Autodesk Inventor part; units mm, degrees
(part 13 of 13)
  line L4684 (16.4485, 3.9123) -> (16.4485, 3.1666)
  arc A4680 (16.4485, 3.1666) -> (16.6009, 3.1666) centre (16.5247, 3.1666) ccw
  line L4685 (16.6009, 3.1666) -> (16.6009, 3.9123)
  arc A4681 (16.6009, 3.9123) -> (16.4485, 3.9123) centre (16.5247, 3.9123) ccw
  line L4686 (16.5247, 3.2428) -> (15.9654, 3.2428)
  arc A4682 (15.9654, 3.2428) -> (15.9654, 3.0904) centre (15.9654, 3.1666) ccw
  line L4687 (15.9654, 3.0904) -> (16.5247, 3.0904)
  arc A4683 (16.5247, 3.0904) -> (16.5247, 3.2428) centre (16.5247, 3.1666) ccw
  line L4688 (16.0335, 3.1325) -> (16.22, 3.5053)
  arc A4684 (16.22, 3.5053) -> (16.0838, 3.5735) centre (16.1519, 3.5394) ccw
  line L4689 (16.0838, 3.5735) -> (15.8973, 3.2007)
  arc A4685 (15.8973, 3.2007) -> (16.0335, 3.1325) centre (15.9654, 3.1666) ccw
  line L4690 (16.2281, 3.5394) -> (16.2281, 3.7258)
  arc A4686 (16.2281, 3.7258) -> (16.0757, 3.7258) centre (16.1519, 3.7258) ccw
  line L4691 (16.0757, 3.7258) -> (16.0757, 3.5394)
  arc A4687 (16.0757, 3.5394) -> (16.2281, 3.5394) centre (16.1519, 3.5394) ccw
  line L4692 (16.2058, 3.7797) -> (16.0193, 3.9662)
  arc A4688 (16.0193, 3.9662) -> (15.9115, 3.8584) centre (15.9654, 3.9123) ccw
  line L4693 (15.9115, 3.8584) -> (16.098, 3.6719)
  arc A4689 (16.098, 3.6719) -> (16.2058, 3.7797) centre (16.1519, 3.7258) ccw
  line L4694 (15.9654, 3.9885) -> (15.5926, 3.9885)
  arc A4690 (15.5926, 3.9885) -> (15.5926, 3.8361) centre (15.5926, 3.9123) ccw
  line L4695 (15.5926, 3.8361) -> (15.9654, 3.8361)
  arc A4691 (15.9654, 3.8361) -> (15.9654, 3.9885) centre (15.9654, 3.9123) ccw
  line L4696 (15.5387, 3.9662) -> (15.3523, 3.7797)
  arc A4692 (15.3523, 3.7797) -> (15.4601, 3.6719) centre (15.4062, 3.7258) ccw
  line L4697 (15.4601, 3.6719) -> (15.6465, 3.8584)
  arc A4693 (15.6465, 3.8584) -> (15.5387, 3.9662) centre (15.5926, 3.9123) ccw
  line L4698 (15.33, 3.7258) -> (15.33, 3.353)
  arc A4694 (15.33, 3.353) -> (15.4824, 3.353) centre (15.4062, 3.353) ccw
  line L4699 (15.4824, 3.353) -> (15.4824, 3.7258)
  arc A4695 (15.4824, 3.7258) -> (15.33, 3.7258) centre (15.4062, 3.7258) ccw
  line L4700 (15.3523, 3.2991) -> (15.5387, 3.1127)
  arc A4696 (15.5387, 3.1127) -> (15.6465, 3.2205) centre (15.5926, 3.1666) ccw
  line L4701 (15.6465, 3.2205) -> (15.4601, 3.4069)
  arc A4697 (15.4601, 3.4069) -> (15.3523, 3.2991) centre (15.4062, 3.353) ccw
  line L4702 (15.4062, 4.2597) -> (16.5247, 4.2597)
  arc A4698 (16.5247, 4.2597) -> (16.5247, 4.4121) centre (16.5247, 4.3359) ccw
  line L4703 (16.5247, 4.4121) -> (15.4062, 4.4121)
  arc A4699 (15.4062, 4.4121) -> (15.4062, 4.2597) centre (15.4062, 4.3359) ccw
  line L4704 (16.5786, 4.3898) -> (16.2058, 4.7626)
  arc A4700 (16.2058, 4.7626) -> (16.098, 4.6548) centre (16.1519, 4.7087) ccw
  line L4705 (16.098, 4.6548) -> (16.4708, 4.282)
  arc A4701 (16.4708, 4.282) -> (16.5786, 4.3898) centre (16.5247, 4.3359) ccw
  line L4706 (16.2058, 4.6548) -> (16.5786, 5.0277)
  arc A4702 (16.5786, 5.0277) -> (16.4708, 5.1355) centre (16.5247, 5.0816) ccw
  line L4707 (16.4708, 5.1355) -> (16.098, 4.7626)
  arc A4703 (16.098, 4.7626) -> (16.2058, 4.6548) centre (16.1519, 4.7087) ccw
  arc A4704 (3.9356, 63.3973) -> (3.8278, 63.5051) centre (3.8817, 63.4512) ccw
  line L4708 (3.8278, 63.5051) -> (3.6414, 63.3186)
  arc A4705 (3.6414, 63.3186) -> (3.7492, 63.2108) centre (3.6953, 63.2647) ccw
  line L4709 (3.8817, 63.375) -> (4.0681, 63.375)
  arc A4706 (4.0681, 63.375) -> (4.0681, 63.5274) centre (4.0681, 63.4512) ccw
  line L4710 (4.0681, 63.5274) -> (3.8817, 63.5274)
  arc A4707 (3.8817, 63.5274) -> (3.8817, 63.375) centre (3.8817, 63.4512) ccw
  line L4711 (4.0142, 63.3973) -> (4.2007, 63.2108)
  arc A4708 (4.2007, 63.2108) -> (4.3085, 63.3186) centre (4.2546, 63.2647) ccw
  line L4712 (4.3085, 63.3186) -> (4.122, 63.5051)
  arc A4709 (4.122, 63.5051) -> (4.0142, 63.3973) centre (4.0681, 63.4512) ccw
  arc A4710 (2.9, 16.9912) -> (2.7476, 16.9912) centre (2.8238, 16.9912) ccw
  arc A4711 (4.1784, 63.0783) -> (4.3308, 63.0783) centre (4.2546, 63.0783) ccw
  line L4713 (4.3308, 63.0783) -> (4.3308, 63.2647)
  arc A4712 (4.3308, 63.2647) -> (4.1784, 63.2647) centre (4.2546, 63.2647) ccw
  line L4714 (4.3085, 63.2108) -> (4.4949, 63.3973)
  arc A4713 (4.4949, 63.3973) -> (4.3871, 63.5051) centre (4.441, 63.4512) ccw
  line L4715 (4.3871, 63.5051) -> (4.2007, 63.3186)
  arc A4714 (4.2007, 63.3186) -> (4.3085, 63.2108) centre (4.2546, 63.2647) ccw
  line L4716 (4.441, 63.375) -> (4.6274, 63.375)
  arc A4715 (4.6274, 63.375) -> (4.6274, 63.5274) centre (4.6274, 63.4512) ccw
  line L4717 (4.6274, 63.5274) -> (4.441, 63.5274)
  arc A4716 (4.441, 63.5274) -> (4.441, 63.375) centre (4.441, 63.4512) ccw
  line L4718 (4.5735, 63.3973) -> (4.7599, 63.2108)
  arc A4717 (4.7599, 63.2108) -> (4.8677, 63.3186) centre (4.8138, 63.2647) ccw
  line L4719 (4.8677, 63.3186) -> (4.6813, 63.5051)
  arc A4718 (4.6813, 63.5051) -> (4.5735, 63.3973) centre (4.6274, 63.4512) ccw
  line L4720 (4.1784, 63.2647) -> (4.1784, 63.0783)
  line L4721 (4.7376, 63.2647) -> (4.7376, 62.8919)
  arc A4719 (4.7376, 62.8919) -> (4.89, 62.8919) centre (4.8138, 62.8919) ccw
  line L4722 (4.89, 62.8919) -> (4.89, 63.2647)
  arc A4720 (4.89, 63.2647) -> (4.7376, 63.2647) centre (4.8138, 63.2647) ccw
  line L4723 (4.7599, 62.9458) -> (4.5735, 62.7594)
  arc A4721 (4.5735, 62.7594) -> (4.6813, 62.6516) centre (4.6274, 62.7055) ccw
  line L4724 (4.6813, 62.6516) -> (4.8677, 62.838)
  arc A4722 (4.8677, 62.838) -> (4.7599, 62.9458) centre (4.8138, 62.8919) ccw
  line L4725 (2.6913, 15.0223) -> (2.8777, 15.2087)
  arc A4723 (2.8777, 15.2087) -> (2.7699, 15.3165) centre (2.8238, 15.2626) ccw
  line L4726 (2.7699, 15.3165) -> (2.5835, 15.1301)
  arc A4724 (2.5835, 15.1301) -> (2.6913, 15.0223) centre (2.6374, 15.0762) ccw
  line L4727 (2.9, 15.2626) -> (2.9, 15.449)
  arc A4725 (2.9, 15.449) -> (2.7476, 15.449) centre (2.8238, 15.449) ccw
  line L4728 (2.7476, 15.449) -> (2.7476, 15.2626)
  arc A4726 (2.7476, 15.2626) -> (2.9, 15.2626) centre (2.8238, 15.2626) ccw
  line L4729 (2.8777, 15.5029) -> (2.6913, 15.6893)
  arc A4727 (2.6913, 15.6893) -> (2.5835, 15.5815) centre (2.6374, 15.6354) ccw
  line L4730 (2.5835, 15.5815) -> (2.7699, 15.3951)
  arc A4728 (2.7699, 15.3951) -> (2.8777, 15.5029) centre (2.8238, 15.449) ccw
  line L4731 (2.6374, 15.7116) -> (1.7053, 15.7116)
  arc A4729 (1.7053, 15.7116) -> (1.7053, 15.5592) centre (1.7053, 15.6354) ccw
  line L4732 (1.7053, 15.5592) -> (2.6374, 15.5592)
  arc A4730 (2.6374, 15.5592) -> (2.6374, 15.7116) centre (2.6374, 15.6354) ccw
  line L4733 (1.7815, 15.449) -> (1.7815, 15.8219)
  arc A4731 (1.7815, 15.8219) -> (1.6291, 15.8219) centre (1.7053, 15.8219) ccw
  line L4734 (1.6291, 15.8219) -> (1.6291, 15.449)
  arc A4732 (1.6291, 15.449) -> (1.7815, 15.449) centre (1.7053, 15.449) ccw
  line L4735 (2.132, 16.2994) -> (1.7592, 16.6722)
  arc A4733 (1.7592, 16.6722) -> (1.6514, 16.5644) centre (1.7053, 16.6183) ccw
  line L4736 (1.6514, 16.5644) -> (2.0242, 16.1916)
  arc A4734 (2.0242, 16.1916) -> (2.132, 16.2994) centre (2.0781, 16.2455) ccw
  line L4737 (1.7053, 16.5421) -> (2.8238, 16.5421)
  arc A4735 (2.8238, 16.5421) -> (2.8238, 16.6945) centre (2.8238, 16.6183) ccw
  line L4738 (2.8238, 16.6945) -> (1.7053, 16.6945)
  arc A4736 (1.7053, 16.6945) -> (1.7053, 16.5421) centre (1.7053, 16.6183) ccw
  line L4739 (2.9, 16.2455) -> (2.9, 16.9912)
  line L4740 (2.7476, 16.9912) -> (2.7476, 16.2455)
  arc A4737 (2.7476, 16.2455) -> (2.9, 16.2455) centre (2.8238, 16.2455) ccw
  line L4741 (4.6813, 61.4823) -> (4.8677, 61.6687)
  arc A4738 (4.8677, 61.6687) -> (4.7599, 61.7765) centre (4.8138, 61.7226) ccw
  line L4742 (4.7599, 61.7765) -> (4.5735, 61.5901)
  arc A4739 (4.5735, 61.5901) -> (4.6813, 61.4823) centre (4.6274, 61.5362) ccw
  line L4743 (4.89, 61.7226) -> (4.89, 61.909)
  arc A4740 (4.89, 61.909) -> (4.7376, 61.909) centre (4.8138, 61.909) ccw
  line L4744 (4.7376, 61.909) -> (4.7376, 61.7226)
  arc A4741 (4.7376, 61.7226) -> (4.89, 61.7226) centre (4.8138, 61.7226) ccw
  line L4745 (4.8677, 61.9629) -> (4.6813, 62.1493)
  arc A4742 (4.6813, 62.1493) -> (4.5735, 62.0415) centre (4.6274, 62.0954) ccw
  line L4746 (4.5735, 62.0415) -> (4.7599, 61.8551)
  arc A4743 (4.7599, 61.8551) -> (4.8677, 61.9629) centre (4.8138, 61.909) ccw
  line L4747 (4.6274, 62.1716) -> (3.6953, 62.1716)
  arc A4744 (3.6953, 62.1716) -> (3.6953, 62.0192) centre (3.6953, 62.0954) ccw
  line L4748 (3.6953, 62.0192) -> (4.6274, 62.0192)
  arc A4745 (4.6274, 62.0192) -> (4.6274, 62.1716) centre (4.6274, 62.0954) ccw
  line L4749 (3.7715, 61.909) -> (3.7715, 62.2819)
  arc A4746 (3.7715, 62.2819) -> (3.6191, 62.2819) centre (3.6953, 62.2819) ccw
  line L4750 (3.6191, 62.2819) -> (3.6191, 61.909)
  arc A4747 (3.6191, 61.909) -> (3.7715, 61.909) centre (3.6953, 61.909) ccw
  line L4751 (3.9356, 62.7594) -> (3.7492, 62.9458)
  arc A4748 (3.7492, 62.9458) -> (3.6414, 62.838) centre (3.6953, 62.8919) ccw
  line L4752 (3.6414, 62.838) -> (3.8278, 62.6516)
  arc A4749 (3.8278, 62.6516) -> (3.9356, 62.7594) centre (3.8817, 62.7055) ccw
  line L4753 (3.7715, 62.8919) -> (3.7715, 63.2647)
  arc A4750 (3.7715, 63.2647) -> (3.6191, 63.2647) centre (3.6953, 63.2647) ccw
  line L4754 (3.6191, 63.2647) -> (3.6191, 62.8919)
  arc A4751 (3.6191, 62.8919) -> (3.7715, 62.8919) centre (3.6953, 62.8919) ccw
  line L4755 (3.7492, 63.2108) -> (3.9356, 63.3973)
  line L4756 (0, 64.2) -> (0, 0)
  line L4757 (18.2, 64.2) -> (0, 64.2)
  line L4758 (18.2, 0) -> (18.2, 64.2)
  line L4759 (0, 0) -> (18.2, 0)
  arc A4752 (7.5476, 4.1362) -> (7.7, 4.1362) centre (7.6238, 4.1362) ccw
  line L4760 (10.0313, 29.4823) -> (10.2177, 29.6687)
  arc A4753 (10.2177, 29.6687) -> (10.1099, 29.7765) centre (10.1638, 29.7226) ccw
  line L4761 (10.1099, 29.7765) -> (9.9235, 29.5901)
  arc A4754 (9.9235, 29.5901) -> (10.0313, 29.4823) centre (9.9774, 29.5362) ccw
  line L4762 (10.24, 29.7226) -> (10.24, 29.909)
  arc A4755 (10.24, 29.909) -> (10.0876, 29.909) centre (10.1638, 29.909) ccw
  line L4763 (10.0876, 29.909) -> (10.0876, 29.7226)
  arc A4756 (10.0876, 29.7226) -> (10.24, 29.7226) centre (10.1638, 29.7226) ccw
  line L4764 (10.2177, 29.9629) -> (10.0313, 30.1493)
  arc A4757 (10.0313, 30.1493) -> (9.9235, 30.0415) centre (9.9774, 30.0954) ccw
  line L4765 (9.9235, 30.0415) -> (10.1099, 29.8551)
  arc A4758 (10.1099, 29.8551) -> (10.2177, 29.9629) centre (10.1638, 29.909) ccw
  line L4766 (9.9774, 30.1716) -> (9.0453, 30.1716)
  arc A4759 (9.0453, 30.1716) -> (9.0453, 30.0192) centre (9.0453, 30.0954) ccw
  line L4767 (9.0453, 30.0192) -> (9.9774, 30.0192)
  arc A4760 (9.9774, 30.0192) -> (9.9774, 30.1716) centre (9.9774, 30.0954) ccw
  line L4768 (9.1215, 29.909) -> (9.1215, 30.2819)
  arc A4761 (9.1215, 30.2819) -> (8.9691, 30.2819) centre (9.0453, 30.2819) ccw
  line L4769 (8.9691, 30.2819) -> (8.9691, 29.909)
  arc A4762 (8.9691, 29.909) -> (9.1215, 29.909) centre (9.0453, 29.909) ccw
  line L4770 (9.2856, 30.7594) -> (9.0992, 30.9458)
  arc A4763 (9.0992, 30.9458) -> (8.9914, 30.838) centre (9.0453, 30.8919) ccw
  arc A4764 (9.1778, 30.6516) -> (9.2856, 30.7594) centre (9.2317, 30.7055) ccw
  line L4771 (9.1215, 30.8919) -> (9.1215, 31.2647)
  arc A4765 (9.1215, 31.2647) -> (8.9691, 31.2647) centre (9.0453, 31.2647) ccw
  line L4772 (8.9691, 31.2647) -> (8.9691, 30.8919)
  arc A4766 (8.9691, 30.8919) -> (9.1215, 30.8919) centre (9.0453, 30.8919) ccw
  line L4773 (9.0992, 31.2108) -> (9.2856, 31.3973)
  arc A4767 (9.2856, 31.3973) -> (9.1778, 31.5051) centre (9.2317, 31.4512) ccw
  line L4774 (9.1778, 31.5051) -> (8.9914, 31.3186)
  arc A4768 (8.9914, 31.3186) -> (9.0992, 31.2108) centre (9.0453, 31.2647) ccw
  line L4775 (9.2317, 31.375) -> (9.4181, 31.375)
  arc A4769 (9.4181, 31.375) -> (9.4181, 31.5274) centre (9.4181, 31.4512) ccw
  line L4776 (9.4181, 31.5274) -> (9.2317, 31.5274)
  arc A4770 (9.2317, 31.5274) -> (9.2317, 31.375) centre (9.2317, 31.4512) ccw
  line L4777 (9.3642, 31.3973) -> (9.5507, 31.2108)
  arc A4771 (9.5507, 31.2108) -> (9.6585, 31.3186) centre (9.6046, 31.2647) ccw
  line L4778 (9.6585, 31.3186) -> (9.472, 31.5051)
  arc A4772 (9.472, 31.5051) -> (9.3642, 31.3973) centre (9.4181, 31.4512) ccw
  line L4779 (9.5284, 31.2647) -> (9.5284, 31.0783)
  arc A4773 (9.5284, 31.0783) -> (9.6808, 31.0783) centre (9.6046, 31.0783) ccw
  line L4780 (9.6808, 31.0783) -> (9.6808, 31.2647)
  arc A4774 (9.6808, 31.2647) -> (9.5284, 31.2647) centre (9.6046, 31.2647) ccw
  line L4781 (9.6585, 31.2108) -> (9.8449, 31.3973)
  arc A4775 (9.8449, 31.3973) -> (9.7371, 31.5051) centre (9.791, 31.4512) ccw
  line L4782 (9.7371, 31.5051) -> (9.5507, 31.3186)
  arc A4776 (9.5507, 31.3186) -> (9.6585, 31.2108) centre (9.6046, 31.2647) ccw
  line L4783 (9.791, 31.375) -> (9.9774, 31.375)
  arc A4777 (9.9774, 31.375) -> (9.9774, 31.5274) centre (9.9774, 31.4512) ccw
  line L4784 (9.9774, 31.5274) -> (9.791, 31.5274)
  arc A4778 (9.791, 31.5274) -> (9.791, 31.375) centre (9.791, 31.4512) ccw
  line L4785 (9.9235, 31.3973) -> (10.1099, 31.2108)
  arc A4779 (10.1099, 31.2108) -> (10.2177, 31.3186) centre (10.1638, 31.2647) ccw
  line L4786 (10.2177, 31.3186) -> (10.0313, 31.5051)
  arc A4780 (10.0313, 31.5051) -> (9.9235, 31.3973) centre (9.9774, 31.4512) ccw
  line L4787 (10.0876, 31.2647) -> (10.0876, 30.8919)
  arc A4781 (10.0876, 30.8919) -> (10.24, 30.8919) centre (10.1638, 30.8919) ccw
  line L4788 (10.24, 30.8919) -> (10.24, 31.2647)
  arc A4782 (10.24, 31.2647) -> (10.0876, 31.2647) centre (10.1638, 31.2647) ccw
  line L4789 (10.1099, 30.9458) -> (9.9235, 30.7594)
  arc A4783 (9.9235, 30.7594) -> (10.0313, 30.6516) centre (9.9774, 30.7055) ccw
  arc A4784 (2.8826, 35.7876) -> (3.035, 35.7876) centre (2.9588, 35.7876) ccw
  line L4790 (3.0127, 36.0279) -> (2.8263, 36.2143)
  arc A4785 (2.8263, 36.2143) -> (2.7185, 36.1065) centre (2.7724, 36.1604) ccw
  line L4791 (2.7185, 36.1065) -> (2.9049, 35.9201)
  arc A4786 (2.9049, 35.9201) -> (3.0127, 36.0279) centre (2.9588, 35.974) ccw
  line L4792 (2.7724, 36.2366) -> (1.8403, 36.2366)
  arc A4787 (1.8403, 36.2366) -> (1.8403, 36.0842) centre (1.8403, 36.1604) ccw
  line L4793 (1.8403, 36.0842) -> (2.7724, 36.0842)
  arc A4788 (2.7724, 36.0842) -> (2.7724, 36.2366) centre (2.7724, 36.1604) ccw
  line L4794 (1.9165, 35.974) -> (1.9165, 36.3469)
  arc A4789 (1.9165, 36.3469) -> (1.7641, 36.3469) centre (1.8403, 36.3469) ccw
  line L4795 (1.7641, 36.3469) -> (1.7641, 35.974)
  arc A4790 (1.7641, 35.974) -> (1.9165, 35.974) centre (1.8403, 35.974) ccw
  line L4796 (2.267, 36.8244) -> (1.8942, 37.1972)
  arc A4791 (1.8942, 37.1972) -> (1.7864, 37.0894) centre (1.8403, 37.1433) ccw
  line L4797 (1.7864, 37.0894) -> (2.1592, 36.7166)
  arc A4792 (2.1592, 36.7166) -> (2.267, 36.8244) centre (2.2131, 36.7705) ccw
  line L4798 (1.8403, 37.0671) -> (2.9588, 37.0671)
  arc A4793 (2.9588, 37.0671) -> (2.9588, 37.2195) centre (2.9588, 37.1433) ccw
  line L4799 (2.9588, 37.2195) -> (1.8403, 37.2195)
  arc A4794 (1.8403, 37.2195) -> (1.8403, 37.0671) centre (1.8403, 37.1433) ccw
  line L4800 (3.035, 36.7705) -> (3.035, 37.5162)
  arc A4795 (3.035, 37.5162) -> (2.8826, 37.5162) centre (2.9588, 37.5162) ccw
  arc A4796 (6.5053, 4.5852) -> (6.5053, 4.4328) centre (6.5053, 4.509) ccw
  line L4801 (1, 59.7) -> (1, 17.7)
  line L4802 (3.035, 35.7876) -> (3.035, 35.974)
  line L4803 (8.9914, 30.838) -> (9.1778, 30.6516)
  arc A4797 (3.035, 35.974) -> (2.8826, 35.974) centre (2.9588, 35.974) ccw
  line L4804 (2.8826, 35.974) -> (2.8826, 35.7876)
  arc A4798 (10.2177, 30.838) -> (10.1099, 30.9458) centre (10.1638, 30.8919) ccw
  line L4805 (5.7, 63.08) -> (17.7, 63.08)
  line L4806 (17.7, 63.08) -> (17.7, 0.92)
  line L4807 (17.7, 0.92) -> (5.7, 0.92)
  line L4808 (5.7, 0.92) -> (5.7, 63.08)
  line L4809 (1, 17.7) -> (3.8, 17.7)
  line L4810 (7.7, 4.1362) -> (7.7, 4.8819)
  arc A4799 (7.7, 4.8819) -> (7.5476, 4.8819) centre (7.6238, 4.8819) ccw
  line L4811 (7.5476, 4.8819) -> (7.5476, 4.1362)
  line L4812 (2.8826, 37.5162) -> (2.8826, 36.7705)
  line L4813 (10.0313, 30.6516) -> (10.2177, 30.838)
  line L4814 (3.8, 17.7) -> (3.8, 59.7)
  line L4815 (3.8, 59.7) -> (1, 59.7)
  line L4816 (2.8263, 35.5473) -> (3.0127, 35.7337)
  arc A4800 (3.0127, 35.7337) -> (2.9049, 35.8415) centre (2.9588, 35.7876) ccw
  line L4817 (2.9049, 35.8415) -> (2.7185, 35.6551)
  arc A4801 (2.7185, 35.6551) -> (2.8263, 35.5473) centre (2.7724, 35.6012) ccw
  line L4818 (6.932, 4.1901) -> (6.5592, 4.5629)
  arc A4802 (6.5592, 4.5629) -> (6.4514, 4.4551) centre (6.5053, 4.509) ccw
  line L4819 (6.4514, 4.4551) -> (6.8242, 4.0823)
  arc A4803 (6.8242, 4.0823) -> (6.932, 4.1901) centre (6.8781, 4.1362) ccw
  line L4820 (6.5053, 4.4328) -> (7.6238, 4.4328)
  arc A4804 (7.6238, 4.4328) -> (7.6238, 4.5852) centre (7.6238, 4.509) ccw
  line L4821 (7.6238, 4.5852) -> (6.5053, 4.5852)
  arc A4805 (2.8826, 36.7705) -> (3.035, 36.7705) centre (2.9588, 36.7705) ccw
  line L4822 (3.3, 18.55) -> (3.3, 20.35)
  line L4823 (3.3, 20.35) -> (1.5, 20.35)
  line L4824 (1.5, 20.35) -> (1.5, 18.55)
  line L4825 (1.5, 18.55) -> (3.3, 18.55)
  line L4826 (3.3, 18.55) -> (3.3, 20.35)
  line L4827 (3.3, 20.35) -> (1.5, 20.35)
  line L4828 (1.5, 20.35) -> (1.5, 18.55)
  line L4829 (1.5, 18.55) -> (3.3, 18.55)
  circle A4806 centre (2.4, 22.95) radius 0.9
  circle A4807 centre (2.4, 22.95) radius 0.9
  circle A4808 centre (2.4, 26.45) radius 0.9
  circle A4809 centre (2.4, 26.45) radius 0.9
  circle A4810 centre (2.4, 29.95) radius 0.9
  circle A4811 centre (2.4, 29.95) radius 0.9
  circle A4812 centre (2.4, 33.45) radius 0.9
  circle A4813 centre (2.4, 33.45) radius 0.9
  circle A4814 centre (2.4, 36.95) radius 0.9
  circle A4815 centre (2.4, 36.95) radius 0.9
  circle A4816 centre (2.4, 40.45) radius 0.9
  circle A4817 centre (2.4, 40.45) radius 0.9
  circle A4818 centre (2.4, 43.95) radius 0.9
  circle A4819 centre (2.4, 43.95) radius 0.9
  circle A4820 centre (2.4, 47.45) radius 0.9
  circle A4821 centre (2.4, 47.45) radius 0.9
  circle A4822 centre (2.4, 50.95) radius 0.9
  circle A4823 centre (2.4, 50.95) radius 0.9
  circle A4824 centre (2.4, 54.45) radius 0.9
  circle A4825 centre (2.4, 54.45) radius 0.9
  circle A4826 centre (2.4, 57.95) radius 0.9
  circle A4827 centre (2.4, 57.95) radius 0.9
  line L4830 (8.75, 3.01) -> (8.75, 5.11)
  line L4831 (8.75, 5.11) -> (6.65, 5.11)
  line L4832 (6.65, 5.11) -> (6.65, 3.01)
  line L4833 (6.65, 3.01) -> (8.75, 3.01)
  line L4834 (8.75, 3.01) -> (8.75, 5.11)
  line L4835 (8.75, 5.11) -> (6.65, 5.11)
  line L4836 (6.65, 5.11) -> (6.65, 3.01)
  line L4837 (6.65, 3.01) -> (8.75, 3.01)
  circle A4828 centre (7.7, 9.14) radius 1.05
  circle A4829 centre (7.7, 9.14) radius 1.05
  circle A4830 centre (7.7, 14.22) radius 1.05
  circle A4831 centre (7.7, 14.22) radius 1.05
  circle A4832 centre (7.7, 19.3) radius 1.05
  circle A4833 centre (7.7, 19.3) radius 1.05
  circle A4834 centre (7.7, 24.38) radius 1.05
  circle A4835 centre (7.7, 24.38) radius 1.05
  circle A4836 centre (7.7, 29.46) radius 1.05
  circle A4837 centre (7.7, 29.46) radius 1.05
  circle A4838 centre (7.7, 34.54) radius 1.05
  circle A4839 centre (7.7, 34.54) radius 1.05
  circle A4840 centre (7.7, 39.62) radius 1.05
  circle A4841 centre (7.7, 39.62) radius 1.05
  circle A4842 centre (7.7, 44.7) radius 1.05
  circle A4843 centre (7.7, 44.7) radius 1.05
  circle A4844 centre (7.7, 49.78) radius 1.05
  circle A4845 centre (7.7, 49.78) radius 1.05
  circle A4846 centre (7.7, 54.86) radius 1.05
  circle A4847 centre (7.7, 54.86) radius 1.05
  circle A4848 centre (7.7, 59.94) radius 1.05
  circle A4849 centre (7.7, 59.94) radius 1.05
  point P0 (7.7, 32)
  point P1 (2.4, 38.7)
  constraints: 10671 point on circle, 9676 end point, 4850 centre point, 918 point on line
sketch "Sketch5" plane through (0, 0, 0) normal (0, 0, 1) x (1, 0, 0)
  line L0 (18.2, 64.2) -> (0, 64.2) projected
  line L1 (18.2, 0) -> (18.2, 64.2) projected
  line L2 (0, 64.2) -> (0, 0) projected
  line L3 (0, 0) -> (18.2, 0) projected
  line L4 (6.65, 3.01) -> (8.75, 3.01) projected
  line L5 (8.75, 3.01) -> (8.75, 5.11) projected
  line L6 (8.75, 5.11) -> (6.65, 5.11) projected
  line L7 (6.65, 5.11) -> (6.65, 3.01) projected
  circle A0 centre (7.7, 9.14) radius 1.05 projected
  circle A1 centre (7.7, 14.22) radius 1.05 projected
  circle A2 centre (7.7, 19.3) radius 1.05 projected
  line L8 (1.5, 18.55) -> (3.3, 18.55) projected
  line L9 (3.3, 18.55) -> (3.3, 20.35) projected
  line L10 (1.5, 20.35) -> (1.5, 18.55) projected
  line L11 (3.3, 20.35) -> (1.5, 20.35) projected
  circle A3 centre (2.4, 22.95) radius 0.9 projected
  circle A4 centre (7.7, 24.38) radius 1.05 projected
  circle A5 centre (2.4, 26.45) radius 0.9 projected
  circle A6 centre (2.4, 29.95) radius 0.9 projected
  circle A7 centre (7.7, 29.46) radius 1.05 projected
  circle A8 centre (7.7, 34.54) radius 1.05 projected
  circle A9 centre (2.4, 33.45) radius 0.9 projected
  circle A10 centre (2.4, 36.95) radius 0.9 projected
  circle A11 centre (7.7, 39.62) radius 1.05 projected
  circle A12 centre (2.4, 40.45) radius 0.9 projected
  circle A13 centre (7.7, 44.7) radius 1.05 projected
  circle A14 centre (2.4, 43.95) radius 0.9 projected
  circle A15 centre (2.4, 47.45) radius 0.9 projected
  circle A16 centre (7.7, 49.78) radius 1.05 projected
  circle A17 centre (2.4, 50.95) radius 0.9 projected
  circle A18 centre (2.4, 54.45) radius 0.9 projected
  circle A19 centre (7.7, 54.86) radius 1.05 projected
  circle A20 centre (2.4, 57.95) radius 0.9 projected
  circle A21 centre (7.7, 59.94) radius 1.05 projected
extrude "Extrusion4" add sketch "Sketch5" along normal blind 1.5748
body "Solid2"
